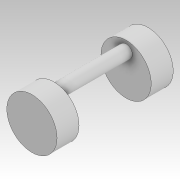
# Autodesk Inventor part: CamShaft
Saved by Autodesk Inventor 2020 (Build 240168000, 168)
## iProperties
Created: 2022-02-03
Part Number: CamShaft
Material: Generic
Document SubType Name: Modeling
Designer: DDeGo
Density: 1 g/cm^3
Appearance: Default
Author: DDeGo
Autodesk Inventor part; units mm, degrees
ref_plane "YZ Plane" through (0, 0, 0) normal (1, 0, 0) x (0, 1, 0)
ref_plane "XZ Plane" through (0, 0, 0) normal (0, 1, 0) x (-1, 0, 0)
ref_plane "XY Plane" through (0, 0, 0) normal (0, 0, 1) x (1, 0, 0)
sketch "Sketch1" plane through (0, 0, 0) normal (0, 0, 1) x (1, 0, 0)
  circle A0 centre (0, 0) radius 4
  dimension "d0" = 8
  constraints: 1 centre point, 1 coincident
  measures "d0" diameter of A0
extrude "Extrusion1" add sketch "Sketch1" along normal blind 3.5
sketch "Sketch2" plane through (0, 0, 0) normal (1, 0, 0) x (0, 1, 0)
  line L0 (4, 0) -> (-4, 0) construction
  line L1 (3.5, 0) -> (3.5, -15)
  line L2 (3.5, -15) -> (2.5, -15)
  line L3 (2.5, -15) -> (2.5, 0)
  line L4 (3.5, 0) -> (2.5, 0)
  line L5 (0, 0) -> (0, -6.9845) construction
  dimension "d3" = 2.5
  dimension "d4" = 1
  dimension "d6" = 15
  constraints: 10 end point, 2 perpendicular, 2 point on line, 2 vertical, 1 collinear
  measures "d3" distance from line of L5.start L3
  measures "d4" distance between parallel lines of L3 L1
  measures "d6" distance of L1.start L1.end
revolve "Revolution1" add sketch "Sketch2" angle 360 about axis through (0, 2.5, -15) along (0, 0, 1)
sketch "Sketch3" plane through (0, 2.5, -15) normal (0, 0, -1) x (-1, 0, 0)
  circle A0 centre (0, -2.5) radius 4 projected
extrude "Extrusion2" add sketch "Sketch3" against normal blind 3.5
body "Solid1"
